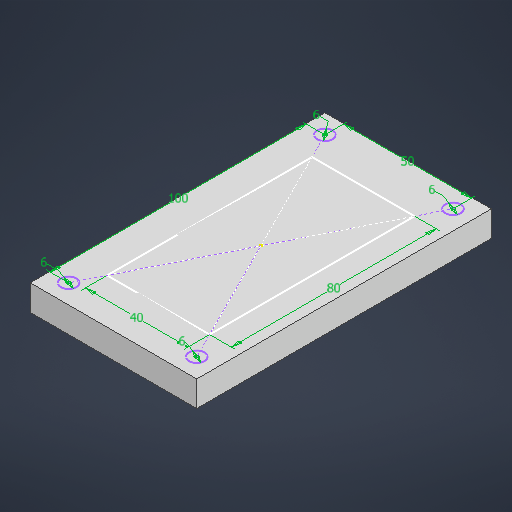
# Autodesk Inventor part: Battery Holder
Saved by Autodesk Inventor 2025 (Build 290162000, 162)
## iProperties
Created: 2025-08-08
Part Number: Battery Holder
Material: Generic
Document SubType Name: Modeling
Designer: mayhe
Density: 1 g/cm^3
Appearance: Default
Author: mayhe
Autodesk Inventor part; units mm, degrees
ref_plane "YZ Plane" through (0, 0, 0) normal (1, 0, 0) x (0, 1, 0)
ref_plane "XZ Plane" through (0, 0, 0) normal (0, 1, 0) x (-1, 0, 0)
ref_plane "XY Plane" through (0, 0, 0) normal (0, 0, 1) x (1, 0, 0)
sketch "Sketch1" plane through (0, 0, 0) normal (0, 1, 0) x (-1, 0, 0)
  line L0 (32.5, 57.5) -> (-32.5, 57.5)
  line L1 (-32.5, 57.5) -> (-32.5, -57.5)
  line L2 (-32.5, -57.5) -> (32.5, -57.5)
  line L3 (32.5, -57.5) -> (32.5, 57.5)
  line L4 (32.5, 57.5) -> (-32.5, -57.5) construction
  line L5 (-32.5, 57.5) -> (32.5, -57.5) construction
  point P0 (0, 0)
  dimension "d0" = 65
  dimension "d1" = 115
  constraints: 12 end point, 2 midpoint, 2 parallel, 1 horizontal, 1 perpendicular
  measures "d0" distance of L2.end L1.end
  measures "d1" distance of L1.end L0.end
extrude "Extrusion1" add sketch "Sketch1" along normal blind 10
sketch "Sketch2" plane through (0, 10, 0) normal (0, 1, 0) x (1, 0, 0)
  line L0 (25, -50) -> (-25, 50) construction
  line L1 (-25, -50) -> (25, 50) construction
  circle A0 centre (25, -50) radius 3
  circle A1 centre (-25, -50) radius 3
  circle A2 centre (25, 50) radius 3
  circle A3 centre (-25, 50) radius 3
  line L2 (-20, 40) -> (20, 40)
  line L3 (20, 40) -> (20, -40)
  line L4 (20, -40) -> (-20, -40)
  line L5 (-20, -40) -> (-20, 40)
  line L6 (-20, 40) -> (20, -40) construction
  line L7 (20, 40) -> (-20, -40) construction
  point P0 (0, 0)
  dimension "d4" = 50
  dimension "d5" = 100
  dimension "d6" = 6
  dimension "d7" = 6
  dimension "d8" = 6
  dimension "d9" = 6
  dimension "d10" = 40
  dimension "d11" = 80
  constraints: 16 end point, 4 centre point, 4 coincident, 4 midpoint, 2 parallel, 1 horizontal, 1 perpendicular
  measures "d4" distance of L0.end L1.end
  measures "d5" distance of L1.start L0.end
  measures "d6" diameter of A0
  measures "d7" diameter of A1
  measures "d8" diameter of A2
  measures "d9" diameter of A3
  measures "d10" distance of L3.end L4.end
  measures "d11" distance of L2.end L3.end
body "Solid1"
